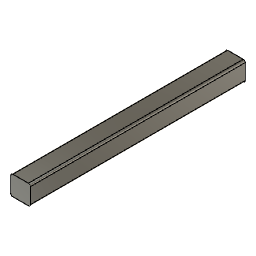
Project Stand Poles v6 (Autodesk Fusion 360 design; units mm, degrees)
Autodesk Fusion 360 part; units mm, degrees
sketch "Sketch1" plane through (0, 0, 0) normal (0, 0, 1) x (1, 0, 0)
  line L0 (-67.3846, 64.3468) -> (-57.8846, 64.3468)
  line L1 (-57.8846, 64.3468) -> (-57.8846, -45.6532)
  line L2 (-57.8846, -45.6532) -> (-67.3846, -45.6532)
  line L3 (-67.3846, -45.6532) -> (-67.3846, 64.3468)
  line L4 (-38.3846, -45.6532) -> (-47.8846, -45.6532)
  line L5 (-38.3846, 64.3468) -> (-38.3846, -45.6532)
  line L6 (-47.8846, -45.6532) -> (-47.8846, 64.3468)
  line L7 (-47.8846, 64.3468) -> (-38.3846, 64.3468)
  line L8 (-18.8846, -45.6532) -> (-28.3846, -45.6532)
  line L9 (-18.8846, 64.3468) -> (-18.8846, -45.6532)
  line L10 (-28.3846, -45.6532) -> (-28.3846, 64.3468)
  line L11 (-28.3846, 64.3468) -> (-18.8846, 64.3468)
  line L12 (0.6154, -45.6532) -> (-8.8846, -45.6532)
  line L13 (0.6154, 64.3468) -> (0.6154, -45.6532)
  line L14 (-8.8846, -45.6532) -> (-8.8846, 64.3468)
  line L15 (-8.8846, 64.3468) -> (0.6154, 64.3468)
  line L16 (20.1154, -45.6532) -> (10.6154, -45.6532)
  line L17 (20.1154, 64.3468) -> (20.1154, -45.6532)
  line L18 (10.6154, -45.6532) -> (10.6154, 64.3468)
  line L19 (10.6154, 64.3468) -> (20.1154, 64.3468)
  line L20 (-77.3846, -45.6532) -> (-87.3846, -45.6532)
  line L21 (-77.3846, 64.3468) -> (-77.3846, -45.6532)
  line L22 (-87.3846, -45.6532) -> (-87.3846, 64.3468)
  line L23 (-87.3846, 64.3468) -> (-77.3846, 64.3468)
  line L24 (-97.3846, 74.3468) -> (30.6154, 74.3468)
  line L25 (30.6154, 74.3468) -> (30.6154, -55.6532)
  line L26 (30.6154, -55.6532) -> (-97.3846, -55.6532)
  line L27 (-97.3846, -55.6532) -> (-97.3846, 74.3468)
  dimension "d1" = 9.5
  dimension "d2" = 110
  dimension "d3" = 9.5
  dimension "d4" = 110
  dimension "d5" = 9.5
  dimension "d6" = 110
  dimension "d7" = 9.5
  dimension "d8" = 110
  dimension "d9" = 9.5
  dimension "d10" = 110
  dimension "d11" = 10
  dimension "d12" = 110
  dimension "d13" = 10
  dimension "d14" = 10
  dimension "d15" = 10
  dimension "d16" = 10
  dimension "d17" = 10
  dimension "d18" = 10
  dimension "d19" = 10
  dimension "d20" = 10
  dimension "d21" = 10
  dimension "d22" = 10
  dimension "d23" = 10
  dimension "d24" = 10
  dimension "d25" = 10
  constraint horizontal L0
  constraint vertical L1
  constraint horizontal L2
  constraint vertical L3
  constraint horizontal L7
  constraint vertical L5
  constraint horizontal L4
  constraint vertical L6
  constraint horizontal L11
  constraint vertical L9
  constraint horizontal L8
  constraint vertical L10
  constraint horizontal L15
  constraint vertical L13
  constraint horizontal L12
  constraint vertical L14
  constraint horizontal L19
  constraint vertical L17
  constraint horizontal L16
  constraint vertical L18
  constraint horizontal L23
  constraint vertical L21
  constraint horizontal L20
  constraint vertical L22
  constraint horizontal L24
  constraint vertical L25
  constraint horizontal L26
  constraint vertical L27
  measures "d1" distance of L0.start L0.end
  measures "d2" distance of L0.start L2.end
  measures "d3" distance of L5.start L6.end
  measures "d4" distance of L6.end L4.end
  measures "d5" distance of L9.start L10.end
  measures "d6" distance of L10.end L8.end
  measures "d7" distance of L13.start L14.end
  measures "d8" distance of L14.end L12.end
  measures "d9" distance of L17.start L18.end
  measures "d10" distance of L18.end L16.end
  measures "d11" distance of L21.start L22.end
  measures "d12" distance of L22.end L20.end
  measures "d13" distance of L23 L24
  measures "d14" distance of L0 L24
  measures "d15" distance of L7 L24
  measures "d16" distance of L11 L24
  measures "d17" distance of L15 L24
  measures "d18" distance of L19 L24
  measures "d19" distance of L20 L26
  measures "d20" distance of L22 L27
  measures "d21" distance of L3 L21
  measures "d22" distance of L1 L6
  measures "d23" distance of L5 L10
  measures "d24" distance of L9 L14
  measures "d25" distance of L13 L18
extrude "Extrude3" add sketch "Sketch1" along normal blind 10 contours L20 L21 L22 L23
fillet "Fillet3" radius 1 2 edges at (-77.3846, 9.3468, 10) (-87.3846, 9.3468, 10)
fillet "Fillet4" radius 1 2 edges at (-77.3846, 9.3468, 0) (-87.3846, 9.3468, 0)
